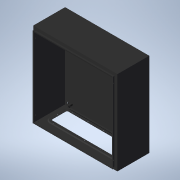
# Autodesk Inventor part: 1054.000(2)_P1
Saved by Autodesk Inventor 2021 (Build 250183000, 183)
## iProperties
Created: 2025-08-26
Part Number: 1054.000(2)_P1
Material: Generic
Catalog Web Link: www.cadenas.de
Description: AE 2.0 Gehaeuse-AE 2.0 Gehaeuse
Vendor: RITTAL
Document SubType Name: Modeling
Designer: psAdmin
Manufacturer: RITTAL
Mass: 1439.52 g
Surface Area: 19061.9 cm^2
Volume: 1439.52 cm^3
Density: 1 g/cm^3
Appearance: PSOLRGB-176-176-176
Category: PARTsolutions
Company: RITTAL
Title: 1054.000(2)_P1
Author: Cadenas PARTsolutions
Comments: AE 2.0 Gehaeuse
PSOL_IDENT_0: {$CADENAS_DATA/23d-libs/rittal/schaltschranksys/kompakt_schaltschr/parts_ae_2_0/gehaeuse_ae_2_0.prj}
PSOL_IDENT_1: ,190 {VTYP=3D},{NB=1054.000(2)_P1},{LINA=1054.000(2)_P1},{NN=AE 2.0 Gehaeuse},{DATE=25.07.2025 12:41
PSOL_IDENT_2: :23},{GEOMDATE=24.07.2025 05:50:00},{VERSION=},{LINEID=340},{WBVAR=DETAIL},{WBNUMERIC=DETAIL}  {NB=1
PSOL_IDENT_3: 054.000(2)_P1},{LINA=1054.000(2)_P1},{KT=DUMMY},{DETAIL=2},{BEZ1=Neues Kompaktgehäuse},{BEZ2=Stahlbl
PSOL_IDENT_4: ech},{BEZ3=eintürig},{TUER=1},{B=600},{H=600},{T=250},{F=550},{G=575},{B1=600},{BEST=1054.000},{B3=5
PSOL_IDENT_5: 60.000},{B4=470.000},{B5=498.000},{BB5=0.000},{H1=600},{H3=560.000},{H4=85.000},{H5=113.000},{HH5=4.
PSOL_IDENT_6: 000},{T5=93.500},{R1=31.000},{R2=8.000},{T1=250},{F1=550},{G1=575},{VERS3=0},{VERS=7},{CNSECLASS51=2
PSOL_IDENT_7: 7-18-01-02},{CNSECLASS70=27-18-01-01},{CNSECLASS80=27-18-01-01},{CNSETIM40=EC000261},{S=1.50},{W=600
PSOL_IDENT_8: .000},{W1=556.000},{W2=500.000},{HH=600.000},{HH1=556.000},{HH2=550.000},{HH3=475.000},{D=227.500},{
PSOL_IDENT_9: D1=245.100},{VERS1=1},{GEW=23,4},{CNSETIM80=EC000261},{CNSETIM90=EC000261},{CNSECLASS60=27-18-01-01}
PSOL_IDENT_10: ,{UNSPSC=31-26-15-02}
NB: 1054.000(2)_P1
NN: AE 2.0 Gehaeuse
NT: AE 2.0 Gehaeuse
NBSYN: $BEST.($DETAIL.)_P1
LINA: 1054.000(2)_P1
CATALOG: Rittal
DETAIL: niedrig
BEZ1: Neues Kompaktgehäuse
BEZ2: Stahlblech
BEZ3: eintürig
TUER: 1
B: 600
H: 600
T: 250
F: 550
G: 575
B1: 600
BEST: 1054.000
B3: 560
B4: 470
B5: 498
BB5: 0
H1: 600
H3: 560
H4: 85
H5: 113
HH5: 4
T5: 93.5
R1: 31
R2: 8
T1: 250
F1: 550
G1: 575
VERS3: 0
VERS: 7
CNSECLASS70: 27-18-01-01
CNSECLASS80: 27-18-01-01
S: 1.5
W: 600
W1: 556
W2: 500
HH: 600
HH1: 556
HH2: 550
HH3: 475
D: 227.5
D1: 245.1
VERS1: 1
GEW: 23,4
CNSETIM80: EC000261
CNSETIM90: EC000261
CNSECLASS60: 27-18-01-01
UNSPSC: 31-26-15-02
SUPPLIER: RITTAL
ARTICLENO: 1054.000(2)_P1
BOMINFO: 1054.000(2)_P1
CREATOR: CADENAS GmbH
Autodesk Inventor part; units mm, degrees
(part 1 of 2)
sketch "Sketch_1" plane through (0, 0, 0) normal (0, 1, 0) x (1, 0, 0)
  line L0 (-300, -102.5) -> (300, -102.5)
  line L1 (300, -102.5) -> (300, 125)
  line L2 (300, 125) -> (-300, 125)
  line L3 (-300, 125) -> (-300, -102.5)
  line L4 (-298.5, -101) -> (298.5, -101)
  line L5 (298.5, -101) -> (298.5, 123.5)
  line L6 (298.5, 123.5) -> (-298.5, 123.5)
  line L7 (-298.5, 123.5) -> (-298.5, -101)
  constraints: 16 end point
extrude "Extrusion1" add sketch "Sketch_1" along normal blind 600
sketch "Sketch_2" plane through (0, 0, 102.5) normal (0, 0, 1) x (1, 0, 0)
  line L0 (-281, 19) -> (281, 19)
  line L1 (281, 19) -> (281, 581)
  line L2 (281, 581) -> (-281, 581)
  line L3 (-281, 581) -> (-281, 19)
  constraints: 8 end point
extrude "Extrusion2" cut sketch "Sketch_2" against normal blind 1.5
sketch "Sketch_3" plane through (0, 0, 0) normal (1, 0, 0) x (0, 0, -1)
  line L0 (-102.5, 590) -> (-101, 590)
  line L1 (-101, 590) -> (-101, 598.5)
  line L2 (-101, 598.5) -> (123.5, 598.5)
  line L3 (123.5, 598.5) -> (123.5, 1.5)
  line L4 (123.5, 1.5) -> (-101, 1.5)
  line L5 (-101, 1.5) -> (-101, 10)
  line L6 (-101, 10) -> (-102.5, 10)
  line L7 (-102.5, 10) -> (-102.5, 0)
  line L8 (-102.5, 0) -> (125, 0)
  line L9 (125, 0) -> (125, 600)
  line L10 (125, 600) -> (-102.5, 600)
  line L11 (-102.5, 600) -> (-102.5, 590)
  constraints: 24 end point
extrude "Extrusion3" add sketch "Sketch_3" along normal mid plane 600
sketch "Sketch_48" plane through (0, 0, -125) normal (0, 0, 1) x (1, 0, 0)
  line L0 (-295.5, 595.5) -> (-295.5, 4.5)
  line L1 (-295.5, 4.5) -> (295.5, 4.5)
  line L2 (295.5, 4.5) -> (295.5, 595.5)
  line L3 (295.5, 595.5) -> (-295.5, 595.5)
  constraints: 8 end point
extrude "Extrusion4" cut sketch "Sketch_48" along normal blind 1.5
sketch "Sketch_49" plane through (0, 0, -125) normal (0, 0, 1) x (1, 0, 0)
  line L0 (-295.5, 595.5) -> (-295.5, 4.5)
  line L1 (-295.5, 4.5) -> (295.5, 4.5)
  line L2 (295.5, 4.5) -> (295.5, 595.5)
  line L3 (295.5, 595.5) -> (-295.5, 595.5)
  line L4 (268.5, 8.5) -> (291.5, 8.5)
  line L5 (291.5, 8.5) -> (291.5, 31.5)
  line L6 (291.5, 31.5) -> (268.5, 31.5)
  line L7 (268.5, 31.5) -> (268.5, 8.5)
  line L8 (268.5, 568.5) -> (291.5, 568.5)
  line L9 (291.5, 568.5) -> (291.5, 591.5)
  line L10 (291.5, 591.5) -> (268.5, 591.5)
  line L11 (268.5, 591.5) -> (268.5, 568.5)
  line L12 (-291.5, 8.5) -> (-268.5, 8.5)
  line L13 (-268.5, 8.5) -> (-268.5, 31.5)
  line L14 (-268.5, 31.5) -> (-291.5, 31.5)
  line L15 (-291.5, 31.5) -> (-291.5, 8.5)
  line L16 (-291.5, 568.5) -> (-268.5, 568.5)
  line L17 (-268.5, 568.5) -> (-268.5, 591.5)
  line L18 (-268.5, 591.5) -> (-291.5, 591.5)
  line L19 (-291.5, 591.5) -> (-291.5, 568.5)
  constraints: 40 end point
extrude "Extrusion5" add sketch "Sketch_49" along normal blind 1.5
sketch "Sketch_50" plane through (0, 20, 0) normal (0, 1, 0) x (1, 0, 0)
  line L0 (-291.5, 123.5) -> (-290.1732, 123.5)
  line L1 (-290.1732, 123.5) -> (-289.0185, 121.5)
  line L2 (-289.0185, 121.5) -> (-270.9815, 121.5)
  line L3 (-270.9815, 121.5) -> (-269.8268, 123.5)
  line L4 (-269.8268, 123.5) -> (-268.5, 123.5)
  line L5 (-268.5, 123.5) -> (-268.5, 125)
  line L6 (-268.5, 125) -> (-270, 125)
  line L7 (-270, 125) -> (-271.1547, 123)
  line L8 (-271.1547, 123) -> (-288.8453, 123)
  line L9 (-288.8453, 123) -> (-290, 125)
  line L10 (-290, 125) -> (-291.5, 125)
  line L11 (-291.5, 125) -> (-291.5, 123.5)
  constraints: 24 end point
extrude "Extrusion6" add sketch "Sketch_50" along normal mid plane 15.35
sketch "Sketch_51" plane through (0, 20, 0) normal (0, 1, 0) x (1, 0, 0)
  line L0 (268.5, 123.5) -> (269.8268, 123.5)
  line L1 (269.8268, 123.5) -> (270.9815, 121.5)
  line L2 (270.9815, 121.5) -> (289.0185, 121.5)
  line L3 (289.0185, 121.5) -> (290.1732, 123.5)
  line L4 (290.1732, 123.5) -> (291.5, 123.5)
  line L5 (291.5, 123.5) -> (291.5, 125)
  line L6 (291.5, 125) -> (290, 125)
  line L7 (290, 125) -> (288.8453, 123)
  line L8 (288.8453, 123) -> (271.1547, 123)
  line L9 (271.1547, 123) -> (270, 125)
  line L10 (270, 125) -> (268.5, 125)
  line L11 (268.5, 125) -> (268.5, 123.5)
  constraints: 24 end point
extrude "Extrusion7" add sketch "Sketch_51" along normal mid plane 15.35
sketch "Sketch_52" plane through (0, 27.675, 0) normal (0, 1, 0) x (1, 0, 0)
  line L0 (-272.325, 121.5) -> (-272.325, 123)
  line L1 (-272.325, 123) -> (-271.1547, 123)
  line L2 (-271.1547, 123) -> (-270, 125)
  line L3 (-270, 125) -> (-265.5, 125)
  line L4 (-265.5, 125) -> (-265.5, 123.5)
  line L5 (-265.5, 123.5) -> (-269.8268, 123.5)
  line L6 (-269.8268, 123.5) -> (-270.9815, 121.5)
  line L7 (-270.9815, 121.5) -> (-272.325, 121.5)
  line L8 (-272.325, 121.5) -> (-272.325, 123)
  constraints: 18 end point
revolve "Revolution1" add sketch "Sketch_52" angle 90 about axis through (-272.325, 27.675, -121.5) along (0, 0, 1)
sketch "Sketch_53" plane through (0, 27.675, 0) normal (0, 1, 0) x (1, 0, 0)
  line L0 (-287.675, 123) -> (-287.675, 121.5)
  line L1 (-287.675, 121.5) -> (-289.0185, 121.5)
  line L2 (-289.0185, 121.5) -> (-290.1732, 123.5)
  line L3 (-290.1732, 123.5) -> (-294.5, 123.5)
  line L4 (-294.5, 123.5) -> (-294.5, 125)
  line L5 (-294.5, 125) -> (-290, 125)
  line L6 (-290, 125) -> (-288.8453, 123)
  line L7 (-288.8453, 123) -> (-287.675, 123)
  line L8 (-287.675, 123) -> (-287.675, 121.5)
  constraints: 18 end point
revolve "Revolution2" add sketch "Sketch_53" angle 90 about axis through (-287.675, 27.675, -123) along (0, 0, -1)
sketch "Sketch_54" plane through (0, 27.675, 0) normal (0, 1, 0) x (1, 0, 0)
  line L0 (287.675, 121.5) -> (287.675, 123)
  line L1 (287.675, 123) -> (288.8453, 123)
  line L2 (288.8453, 123) -> (290, 125)
  line L3 (290, 125) -> (294.5, 125)
  line L4 (294.5, 125) -> (294.5, 123.5)
  line L5 (294.5, 123.5) -> (290.1732, 123.5)
  line L6 (290.1732, 123.5) -> (289.0185, 121.5)
  line L7 (289.0185, 121.5) -> (287.675, 121.5)
  line L8 (287.675, 121.5) -> (287.675, 123)
  constraints: 18 end point
revolve "Revolution3" add sketch "Sketch_54" angle 90 about axis through (287.675, 27.675, -121.5) along (0, 0, 1)
sketch "Sketch_55" plane through (0, 27.675, 0) normal (0, 1, 0) x (1, 0, 0)
  line L0 (272.325, 123) -> (272.325, 121.5)
  line L1 (272.325, 121.5) -> (270.9815, 121.5)
  line L2 (270.9815, 121.5) -> (269.8268, 123.5)
  line L3 (269.8268, 123.5) -> (265.5, 123.5)
  line L4 (265.5, 123.5) -> (265.5, 125)
  line L5 (265.5, 125) -> (270, 125)
  line L6 (270, 125) -> (271.1547, 123)
  line L7 (271.1547, 123) -> (272.325, 123)
  line L8 (272.325, 123) -> (272.325, 121.5)
  constraints: 18 end point
revolve "Revolution4" add sketch "Sketch_55" angle 90 about axis through (272.325, 27.675, -123) along (0, 0, -1)
sketch "Sketch_56" plane through (0, 12.325, 0) normal (0, 1, 0) x (1, 0, 0)
  line L0 (-272.325, 121.5) -> (-272.325, 123)
  line L1 (-272.325, 123) -> (-271.1547, 123)
  line L2 (-271.1547, 123) -> (-270, 125)
  line L3 (-270, 125) -> (-265.5, 125)
  line L4 (-265.5, 125) -> (-265.5, 123.5)
  line L5 (-265.5, 123.5) -> (-269.8268, 123.5)
  line L6 (-269.8268, 123.5) -> (-270.9815, 121.5)
  line L7 (-270.9815, 121.5) -> (-272.325, 121.5)
  line L8 (-272.325, 121.5) -> (-272.325, 123)
  constraints: 18 end point
revolve "Revolution5" add sketch "Sketch_56" angle 90 about axis through (-272.325, 12.325, -121.5) along (0, 0, -1)
sketch "Sketch_57" plane through (0, 12.325, 0) normal (0, 1, 0) x (1, 0, 0)
  line L0 (-287.675, 123) -> (-287.675, 121.5)
  line L1 (-287.675, 121.5) -> (-289.0185, 121.5)
  line L2 (-289.0185, 121.5) -> (-290.1732, 123.5)
  line L3 (-290.1732, 123.5) -> (-294.5, 123.5)
  line L4 (-294.5, 123.5) -> (-294.5, 125)
  line L5 (-294.5, 125) -> (-290, 125)
  line L6 (-290, 125) -> (-288.8453, 123)
  line L7 (-288.8453, 123) -> (-287.675, 123)
  line L8 (-287.675, 123) -> (-287.675, 121.5)
  constraints: 18 end point
revolve "Revolution6" add sketch "Sketch_57" angle 90 about axis through (-287.675, 12.325, -123) along (0, 0, 1)
sketch "Sketch_58" plane through (0, 12.325, 0) normal (0, 1, 0) x (1, 0, 0)
  line L0 (287.675, 121.5) -> (287.675, 123)
  line L1 (287.675, 123) -> (288.8453, 123)
  line L2 (288.8453, 123) -> (290, 125)
  line L3 (290, 125) -> (294.5, 125)
  line L4 (294.5, 125) -> (294.5, 123.5)
  line L5 (294.5, 123.5) -> (290.1732, 123.5)
  line L6 (290.1732, 123.5) -> (289.0185, 121.5)
  line L7 (289.0185, 121.5) -> (287.675, 121.5)
  line L8 (287.675, 121.5) -> (287.675, 123)
  constraints: 18 end point
revolve "Revolution7" add sketch "Sketch_58" angle 90 about axis through (287.675, 12.325, -121.5) along (0, 0, -1)
sketch "Sketch_59" plane through (0, 12.325, 0) normal (0, 1, 0) x (1, 0, 0)
  line L0 (272.325, 123) -> (272.325, 121.5)
  line L1 (272.325, 121.5) -> (270.9815, 121.5)
  line L2 (270.9815, 121.5) -> (269.8268, 123.5)
  line L3 (269.8268, 123.5) -> (265.5, 123.5)
  line L4 (265.5, 123.5) -> (265.5, 125)
  line L5 (265.5, 125) -> (270, 125)
  line L6 (270, 125) -> (271.1547, 123)
  line L7 (271.1547, 123) -> (272.325, 123)
  line L8 (272.325, 123) -> (272.325, 121.5)
  constraints: 18 end point
revolve "Revolution8" add sketch "Sketch_59" angle 90 about axis through (272.325, 12.325, -123) along (0, 0, 1)
sketch "Sketch_60" plane through (0, 580, 0) normal (0, 1, 0) x (1, 0, 0)
  line L0 (-291.5, 123.5) -> (-290.1732, 123.5)
  line L1 (-290.1732, 123.5) -> (-289.0185, 121.5)
  line L2 (-289.0185, 121.5) -> (-270.9815, 121.5)
  line L3 (-270.9815, 121.5) -> (-269.8268, 123.5)
  line L4 (-269.8268, 123.5) -> (-268.5, 123.5)
  line L5 (-268.5, 123.5) -> (-268.5, 125)
  line L6 (-268.5, 125) -> (-270, 125)
  line L7 (-270, 125) -> (-271.1547, 123)
  line L8 (-271.1547, 123) -> (-288.8453, 123)
  line L9 (-288.8453, 123) -> (-290, 125)
  line L10 (-290, 125) -> (-291.5, 125)
  line L11 (-291.5, 125) -> (-291.5, 123.5)
  constraints: 24 end point
extrude "Extrusion8" add sketch "Sketch_60" along normal mid plane 15.35
sketch "Sketch_61" plane through (0, 580, 0) normal (0, 1, 0) x (1, 0, 0)
  line L0 (268.5, 123.5) -> (269.8268, 123.5)
  line L1 (269.8268, 123.5) -> (270.9815, 121.5)
  line L2 (270.9815, 121.5) -> (289.0185, 121.5)
  line L3 (289.0185, 121.5) -> (290.1732, 123.5)
  line L4 (290.1732, 123.5) -> (291.5, 123.5)
  line L5 (291.5, 123.5) -> (291.5, 125)
  line L6 (291.5, 125) -> (290, 125)
  line L7 (290, 125) -> (288.8453, 123)
  line L8 (288.8453, 123) -> (271.1547, 123)
  line L9 (271.1547, 123) -> (270, 125)
  line L10 (270, 125) -> (268.5, 125)
  line L11 (268.5, 125) -> (268.5, 123.5)
  constraints: 24 end point
extrude "Extrusion9" add sketch "Sketch_61" along normal mid plane 15.35
sketch "Sketch_62" plane through (0, 587.675, 0) normal (0, 1, 0) x (1, 0, 0)
  line L0 (-272.325, 121.5) -> (-272.325, 123)
  line L1 (-272.325, 123) -> (-271.1547, 123)
  line L2 (-271.1547, 123) -> (-270, 125)
  line L3 (-270, 125) -> (-265.5, 125)
  line L4 (-265.5, 125) -> (-265.5, 123.5)
  line L5 (-265.5, 123.5) -> (-269.8268, 123.5)
  line L6 (-269.8268, 123.5) -> (-270.9815, 121.5)
  line L7 (-270.9815, 121.5) -> (-272.325, 121.5)
  line L8 (-272.325, 121.5) -> (-272.325, 123)
  constraints: 18 end point
revolve "Revolution9" add sketch "Sketch_62" angle 90 about axis through (-272.325, 587.675, -121.5) along (0, 0, 1)
sketch "Sketch_63" plane through (0, 587.675, 0) normal (0, 1, 0) x (1, 0, 0)
  line L0 (-287.675, 123) -> (-287.675, 121.5)
  line L1 (-287.675, 121.5) -> (-289.0185, 121.5)
  line L2 (-289.0185, 121.5) -> (-290.1732, 123.5)
  line L3 (-290.1732, 123.5) -> (-294.5, 123.5)
  line L4 (-294.5, 123.5) -> (-294.5, 125)
  line L5 (-294.5, 125) -> (-290, 125)
  line L6 (-290, 125) -> (-288.8453, 123)
  line L7 (-288.8453, 123) -> (-287.675, 123)
  line L8 (-287.675, 123) -> (-287.675, 121.5)
  constraints: 18 end point
revolve "Revolution10" add sketch "Sketch_63" angle 90 about axis through (-287.675, 587.675, -123) along (0, 0, -1)
sketch "Sketch_64" plane through (0, 587.675, 0) normal (0, 1, 0) x (1, 0, 0)
  line L0 (287.675, 121.5) -> (287.675, 123)
  line L1 (287.675, 123) -> (288.8453, 123)
  line L2 (288.8453, 123) -> (290, 125)
  line L3 (290, 125) -> (294.5, 125)
  line L4 (294.5, 125) -> (294.5, 123.5)
  line L5 (294.5, 123.5) -> (290.1732, 123.5)
  line L6 (290.1732, 123.5) -> (289.0185, 121.5)
  line L7 (289.0185, 121.5) -> (287.675, 121.5)
  line L8 (287.675, 121.5) -> (287.675, 123)
  constraints: 18 end point
revolve "Revolution11" add sketch "Sketch_64" angle 90 about axis through (287.675, 587.675, -121.5) along (0, 0, 1)
sketch "Sketch_65" plane through (0, 587.675, 0) normal (0, 1, 0) x (1, 0, 0)
  line L0 (272.325, 123) -> (272.325, 121.5)
  line L1 (272.325, 121.5) -> (270.9815, 121.5)
  line L2 (270.9815, 121.5) -> (269.8268, 123.5)
  line L3 (269.8268, 123.5) -> (265.5, 123.5)
  line L4 (265.5, 123.5) -> (265.5, 125)
  line L5 (265.5, 125) -> (270, 125)
  line L6 (270, 125) -> (271.1547, 123)
  line L7 (271.1547, 123) -> (272.325, 123)
  line L8 (272.325, 123) -> (272.325, 121.5)
  constraints: 18 end point
revolve "Revolution12" add sketch "Sketch_65" angle 90 about axis through (272.325, 587.675, -123) along (0, 0, -1)
sketch "Sketch_66" plane through (0, 572.325, 0) normal (0, 1, 0) x (1, 0, 0)
  line L0 (-272.325, 121.5) -> (-272.325, 123)
  line L1 (-272.325, 123) -> (-271.1547, 123)
  line L2 (-271.1547, 123) -> (-270, 125)
  line L3 (-270, 125) -> (-265.5, 125)
  line L4 (-265.5, 125) -> (-265.5, 123.5)
  line L5 (-265.5, 123.5) -> (-269.8268, 123.5)
  line L6 (-269.8268, 123.5) -> (-270.9815, 121.5)
  line L7 (-270.9815, 121.5) -> (-272.325, 121.5)
  line L8 (-272.325, 121.5) -> (-272.325, 123)
  constraints: 18 end point
revolve "Revolution13" add sketch "Sketch_66" angle 90 about axis through (-272.325, 572.325, -121.5) along (0, 0, -1)
sketch "Sketch_67" plane through (0, 572.325, 0) normal (0, 1, 0) x (1, 0, 0)
  line L0 (-287.675, 123) -> (-287.675, 121.5)
  line L1 (-287.675, 121.5) -> (-289.0185, 121.5)
  line L2 (-289.0185, 121.5) -> (-290.1732, 123.5)
  line L3 (-290.1732, 123.5) -> (-294.5, 123.5)
  line L4 (-294.5, 123.5) -> (-294.5, 125)
  line L5 (-294.5, 125) -> (-290, 125)
  line L6 (-290, 125) -> (-288.8453, 123)
  line L7 (-288.8453, 123) -> (-287.675, 123)
  line L8 (-287.675, 123) -> (-287.675, 121.5)
  constraints: 18 end point
revolve "Revolution14" add sketch "Sketch_67" angle 90 about axis through (-287.675, 572.325, -123) along (0, 0, 1)
sketch "Sketch_68" plane through (0, 572.325, 0) normal (0, 1, 0) x (1, 0, 0)
  line L0 (287.675, 121.5) -> (287.675, 123)
  line L1 (287.675, 123) -> (288.8453, 123)
  line L2 (288.8453, 123) -> (290, 125)
  line L3 (290, 125) -> (294.5, 125)
  line L4 (294.5, 125) -> (294.5, 123.5)
  line L5 (294.5, 123.5) -> (290.1732, 123.5)
  line L6 (290.1732, 123.5) -> (289.0185, 121.5)
  line L7 (289.0185, 121.5) -> (287.675, 121.5)
  line L8 (287.675, 121.5) -> (287.675, 123)
  constraints: 18 end point
revolve "Revolution15" add sketch "Sketch_68" angle 90 about axis through (287.675, 572.325, -121.5) along (0, 0, -1)
sketch "Sketch_69" plane through (0, 572.325, 0) normal (0, 1, 0) x (1, 0, 0)
  line L0 (272.325, 123) -> (272.325, 121.5)
  line L1 (272.325, 121.5) -> (270.9815, 121.5)
  line L2 (270.9815, 121.5) -> (269.8268, 123.5)
  line L3 (269.8268, 123.5) -> (265.5, 123.5)
  line L4 (265.5, 123.5) -> (265.5, 125)
  line L5 (265.5, 125) -> (270, 125)
  line L6 (270, 125) -> (271.1547, 123)
  line L7 (271.1547, 123) -> (272.325, 123)
  line L8 (272.325, 123) -> (272.325, 121.5)
  constraints: 18 end point
revolve "Revolution16" add sketch "Sketch_69" angle 90 about axis through (272.325, 572.325, -123) along (0, 0, 1)
sketch "Sketch_70" plane through (-280, 0, 0) normal (1, 0, 0) x (0, 0, -1)
  line L0 (121.5, 10.9815) -> (123.5, 9.8268)
  line L1 (123.5, 9.8268) -> (123.5, 8.5)
  line L2 (123.5, 8.5) -> (125, 8.5)
  line L3 (125, 8.5) -> (125, 10)
  line L4 (125, 10) -> (123, 11.1547)
  line L5 (123, 11.1547) -> (123, 28.8453)
  line L6 (123, 28.8453) -> (125, 30)
  line L7 (125, 30) -> (125, 31.5)
  line L8 (125, 31.5) -> (123.5, 31.5)
  line L9 (123.5, 31.5) -> (123.5, 30.1732)
  line L10 (123.5, 30.1732) -> (121.5, 29.0185)
  line L11 (121.5, 29.0185) -> (121.5, 10.9815)
  constraints: 24 end point
extrude "Extrusion10" add sketch "Sketch_70" along normal mid plane 15.35
sketch "Sketch_71" plane through (-280, 0, 0) normal (1, 0, 0) x (0, 0, -1)
  line L0 (121.5, 570.9815) -> (123.5, 569.8268)
  line L1 (123.5, 569.8268) -> (123.5, 568.5)
  line L2 (123.5, 568.5) -> (125, 568.5)
  line L3 (125, 568.5) -> (125, 570)
  line L4 (125, 570) -> (123, 571.1547)
  line L5 (123, 571.1547) -> (123, 588.8453)
  line L6 (123, 588.8453) -> (125, 590)
  line L7 (125, 590) -> (125, 591.5)
  line L8 (125, 591.5) -> (123.5, 591.5)
  line L9 (123.5, 591.5) -> (123.5, 590.1732)
  line L10 (123.5, 590.1732) -> (121.5, 589.0185)
  line L11 (121.5, 589.0185) -> (121.5, 570.9815)
  constraints: 24 end point
extrude "Extrusion11" add sketch "Sketch_71" along normal mid plane 15.35
sketch "Sketch_74" plane through (-280, 0, 0) normal (1, 0, 0) x (0, 0, -1)
  line L0 (124.5, 20) -> (121.5, 20)
  line L1 (121.5, 20) -> (121.5, 26.25)
  line L2 (121.5, 26.25) -> (123, 26.25)
  line L3 (123, 26.25) -> (123, 25.6)
  line L4 (123, 25.6) -> (124.5, 25.6)
  line L5 (124.5, 25.6) -> (124.5, 20)
  line L6 (124.5, 20) -> (121.5, 20)
  constraints: 14 end point
revolve "Revolution17" add sketch "Sketch_74" angle 360 about axis through (-280, 20, -124.5) along (0, 0, 1)
sketch "Sketch_75" plane through (-280, 0, 0) normal (1, 0, 0) x (0, 0, -1)
  line L0 (125, 20) -> (121, 20)
  line L1 (121, 20) -> (121, 25.625)
  line L2 (121, 25.625) -> (121.5, 25.625)
  line L3 (121.5, 25.625) -> (121.5, 24.625)
  line L4 (121.5, 24.625) -> (124.5, 24.625)
  line L5 (124.5, 24.625) -> (124.5, 25.625)
  line L6 (124.5, 25.625) -> (125, 25.625)
  line L7 (125, 25.625) -> (125, 20)
  line L8 (125, 20) -> (121, 20)
  constraints: 18 end point
revolve "Revolution18" cut sketch "Sketch_75" angle 360 about axis through (-280, 20, -125) along (0, 0, 1)
sketch "Sketch_76" plane through (-280, 0, 0) normal (1, 0, 0) x (0, 0, -1)
  line L0 (124.5, 580) -> (121.5, 580)
  line L1 (121.5, 580) -> (121.5, 586.25)
  line L2 (121.5, 586.25) -> (123, 586.25)
  line L3 (123, 586.25) -> (123, 585.6)
  line L4 (123, 585.6) -> (124.5, 585.6)
  line L5 (124.5, 585.6) -> (124.5, 580)
  line L6 (124.5, 580) -> (121.5, 580)
  constraints: 14 end point
revolve "Revolution19" add sketch "Sketch_76" angle 360 about axis through (-280, 580, -124.5) along (0, 0, 1)
sketch "Sketch_77" plane through (-280, 0, 0) normal (1, 0, 0) x (0, 0, -1)
  line L0 (125, 580) -> (121, 580)
  line L1 (121, 580) -> (121, 585.625)
  line L2 (121, 585.625) -> (121.5, 585.625)
  line L3 (121.5, 585.625) -> (121.5, 584.625)
  line L4 (121.5, 584.625) -> (124.5, 584.625)
  line L5 (124.5, 584.625) -> (124.5, 585.625)
  line L6 (124.5, 585.625) -> (125, 585.625)
  line L7 (125, 585.625) -> (125, 580)
  line L8 (125, 580) -> (121, 580)
  constraints: 18 end point
revolve "Revolution20" cut sketch "Sketch_77" angle 360 about axis through (-280, 580, -125) along (0, 0, 1)
sketch "Sketch_72" plane through (280, 0, 0) normal (1, 0, 0) x (0, 0, -1)
  line L0 (121.5, 10.9815) -> (123.5, 9.8268)
  line L1 (123.5, 9.8268) -> (123.5, 8.5)
  line L2 (123.5, 8.5) -> (125, 8.5)
  line L3 (125, 8.5) -> (125, 10)
  line L4 (125, 10) -> (123, 11.1547)
  line L5 (123, 11.1547) -> (123, 28.8453)
  line L6 (123, 28.8453) -> (125, 30)
  line L7 (125, 30) -> (125, 31.5)
  line L8 (125, 31.5) -> (123.5, 31.5)
  line L9 (123.5, 31.5) -> (123.5, 30.1732)
  line L10 (123.5, 30.1732) -> (121.5, 29.0185)
  line L11 (121.5, 29.0185) -> (121.5, 10.9815)
  constraints: 24 end point
extrude "Extrusion12" add sketch "Sketch_72" along normal mid plane 15.35
sketch "Sketch_73" plane through (280, 0, 0) normal (1, 0, 0) x (0, 0, -1)
  line L0 (121.5, 570.9815) -> (123.5, 569.8268)
  line L1 (123.5, 569.8268) -> (123.5, 568.5)
  line L2 (123.5, 568.5) -> (125, 568.5)
  line L3 (125, 568.5) -> (125, 570)
  line L4 (125, 570) -> (123, 571.1547)
  line L5 (123, 571.1547) -> (123, 588.8453)
  line L6 (123, 588.8453) -> (125, 590)
  line L7 (125, 590) -> (125, 591.5)
  line L8 (125, 591.5) -> (123.5, 591.5)
  line L9 (123.5, 591.5) -> (123.5, 590.1732)
  line L10 (123.5, 590.1732) -> (121.5, 589.0185)
  line L11 (121.5, 589.0185) -> (121.5, 570.9815)
  constraints: 24 end point
extrude "Extrusion13" add sketch "Sketch_73" along normal mid plane 15.35
sketch "Sketch_78" plane through (280, 0, 0) normal (1, 0, 0) x (0, 0, -1)
  line L0 (124.5, 20) -> (121.5, 20)
  line L1 (121.5, 20) -> (121.5, 26.25)
  line L2 (121.5, 26.25) -> (123, 26.25)
  line L3 (123, 26.25) -> (123, 25.6)
  line L4 (123, 25.6) -> (124.5, 25.6)
  line L5 (124.5, 25.6) -> (124.5, 20)
  line L6 (124.5, 20) -> (121.5, 20)
  constraints: 14 end point
revolve "Revolution21" add sketch "Sketch_78" angle 360 about axis through (280, 20, -124.5) along (0, 0, 1)
sketch "Sketch_79" plane through (280, 0, 0) normal (1, 0, 0) x (0, 0, -1)
  line L0 (125, 20) -> (121, 20)
  line L1 (121, 20) -> (121, 25.625)
  line L2 (121, 25.625) -> (121.5, 25.625)
  line L3 (121.5, 25.625) -> (121.5, 24.625)
  line L4 (121.5, 24.625) -> (124.5, 24.625)
  line L5 (124.5, 24.625) -> (124.5, 25.625)
  line L6 (124.5, 25.625) -> (125, 25.625)
  line L7 (125, 25.625) -> (125, 20)
  line L8 (125, 20) -> (121, 20)
  constraints: 18 end point
revolve "Revolution22" cut sketch "Sketch_79" angle 360 about axis through (280, 20, -125) along (0, 0, 1)
sketch "Sketch_80" plane through (280, 0, 0) normal (1, 0, 0) x (0, 0, -1)
  line L0 (124.5, 580) -> (121.5, 580)
  line L1 (121.5, 580) -> (121.5, 586.25)
  line L2 (121.5, 586.25) -> (123, 586.25)
  line L3 (123, 586.25) -> (123, 585.6)
  line L4 (123, 585.6) -> (124.5, 585.6)
  line L5 (124.5, 585.6) -> (124.5, 580)
  line L6 (124.5, 580) -> (121.5, 580)
  constraints: 14 end point
revolve "Revolution23" add sketch "Sketch_80" angle 360 about axis through (280, 580, -124.5) along (0, 0, 1)
sketch "Sketch_81" plane through (280, 0, 0) normal (1, 0, 0) x (0, 0, -1)
  line L0 (125, 580) -> (121, 580)
  line L1 (121, 580) -> (121, 585.625)
  line L2 (121, 585.625) -> (121.5, 585.625)
  line L3 (121.5, 585.625) -> (121.5, 584.625)
  line L4 (121.5, 584.625) -> (124.5, 584.625)
  line L5 (124.5, 584.625) -> (124.5, 585.625)
  line L6 (124.5, 585.625) -> (125, 585.625)
  line L7 (125, 585.625) -> (125, 580)
  line L8 (125, 580) -> (121, 580)
  constraints: 18 end point
revolve "Revolution24" cut sketch "Sketch_81" angle 360 about axis through (280, 580, -125) along (0, 0, 1)
sketch "Sketch_6" plane through (0, 0, 0) normal (1, 0, 0) x (0, 0, -1)
  line L0 (-120.1, 585.9693) -> (-119.4028, 578)
  line L1 (-119.4028, 578) -> (-101, 578)
  line L2 (-101, 578) -> (-101, 586.1)
  line L3 (-101, 586.1) -> (-118.6057, 586.1)
  line L4 (-118.6057, 586.1) -> (-120.1, 585.9693)
  constraints: 10 end point
extrude "Extrusion14" add sketch "Sketch_6" along normal mid plane 574.2
sketch "Sketch_7" plane through (0, 0, 0) normal (1, 0, 0) x (0, 0, -1)
  line L0 (-120.1, 14.0307) -> (-118.6057, 13.9)
  line L1 (-118.6057, 13.9) -> (-101, 13.9)
  line L2 (-101, 13.9) -> (-101, 22)
  line L3 (-101, 22) -> (-119.4028, 22)
  line L4 (-119.4028, 22) -> (-120.1, 14.0307)
  constraints: 10 end point
extrude "Extrusion15" add sketch "Sketch_7" along normal mid plane 574.2
sketch "Sketch_8" plane through (0, 300, 0) normal (0, 1, 0) x (1, 0, 0)
  line L0 (278, -119.4028) -> (285.9693, -120.1)
  line L1 (285.9693, -120.1) -> (286.1, -118.6057)
  line L2 (286.1, -118.6057) -> (286.1, -101)
  line L3 (286.1, -101) -> (278, -101)
  line L4 (278, -101) -> (278, -119.4028)
  constraints: 10 end point
extrude "Extrusion16" add sketch "Sketch_8" along normal mid plane 574.2
sketch "Sketch_9" plane through (0, 300, 0) normal (0, 1, 0) x (1, 0, 0)
  line L0 (-286.1, -118.6057) -> (-285.9693, -120.1)
  line L1 (-285.9693, -120.1) -> (-278, -119.4028)
  line L2 (-278, -119.4028) -> (-278, -101)
  line L3 (-278, -101) -> (-286.1, -101)
  line L4 (-286.1, -101) -> (-286.1, -118.6057)
  constraints: 10 end point
extrude "Extrusion17" add sketch "Sketch_9" along normal mid plane 574.2
sketch "Sketch_10" plane through (0, 300, 0) normal (0, 1, 0) x (1, 0, 0)
  line L0 (-287.6, -102.5) -> (-287.6, -123.1)
  line L1 (-287.6, -123.1) -> (287.6, -123.1)
  line L2 (287.6, -123.1) -> (287.6, -102.5)
  line L3 (287.6, -102.5) -> (279.5, -102.5)
  line L4 (279.5, -102.5) -> (279.5, -118.0283)
  line L5 (279.5, -118.0283) -> (286.1, -118.6057)
  line L6 (286.1, -118.6057) -> (285.9693, -120.1)
  line L7 (285.9693, -120.1) -> (-285.9693, -120.1)
  line L8 (-285.9693, -120.1) -> (-286.1, -118.6057)
  line L9 (-286.1, -118.6057) -> (-279.5, -118.0283)
  line L10 (-279.5, -118.0283) -> (-279.5, -102.5)
  line L11 (-279.5, -102.5) -> (-287.6, -102.5)
  constraints: 24 end point
extrude "Extrusion18" cut sketch "Sketch_10" along normal mid plane 572.2
sketch "Sketch_11" plane through (0, 0, 0) normal (1, 0, 0) x (0, 0, -1)
  line L0 (-123.1, 10.9) -> (-102.5, 10.9)
  line L1 (-102.5, 10.9) -> (-102.5, 20.5)
  line L2 (-102.5, 20.5) -> (-118.0283, 20.5)
  line L3 (-118.0283, 20.5) -> (-118.6057, 13.9)
  line L4 (-118.6057, 13.9) -> (-120.1, 14.0307)
  line L5 (-120.1, 14.0307) -> (-120.1, 585.9693)
  line L6 (-120.1, 585.9693) -> (-118.6057, 586.1)
  line L7 (-118.6057, 586.1) -> (-118.0283, 579.5)
  line L8 (-118.0283, 579.5) -> (-102.5, 579.5)
  line L9 (-102.5, 579.5) -> (-102.5, 589.1)
  line L10 (-102.5, 589.1) -> (-123.1, 589.1)
  line L11 (-123.1, 589.1) -> (-123.1, 10.9)
  constraints: 24 end point
extrude "Extrusion19" cut sketch "Sketch_11" along normal mid plane 572.2
sketch "Sketch_13" plane through (0, 575, 0) normal (0, 1, 0) x (1, 0, 0)
  line L0 (-250, 92.5) -> (-250, 123.5)
  line L1 (-250, 123.5) -> (-243.5, 123.5)
  line L2 (-243.5, 123.5) -> (-243.5, 122.5)
  line L3 (-243.5, 122.5) -> (-242.45, 122.5)
  line L4 (-242.45, 122.5) -> (-242.25, 122.3)
  line L5 (-242.25, 122.3) -> (-242.25, 113.3)
  arc A0 (-242.55, 113) -> (-242.25, 113.3) centre (-242.55, 113.3) ccw
  line L6 (-242.55, 113) -> (-242.25, 113)
  line L7 (-242.25, 113) -> (-242.25, 107.5)
  line L8 (-242.25, 107.5) -> (-246, 107.5)
  line L9 (-246, 107.5) -> (-246, 105)
  line L10 (-246, 105) -> (-241, 105)
  arc A1 (-240.8875, 102.5051) -> (-241, 105) centre (-241, 103.75) ccw
  line L11 (-240.8875, 102.5051) -> (-242.2, 102.3864)
  line L12 (-242.2, 102.3864) -> (-242.2, 97.3483)
  line L13 (-242.2, 97.3483) -> (-243.5, 97)
  line L14 (-243.5, 97) -> (-246, 97)
  line L15 (-246, 97) -> (-246, 93.267)
  line L16 (-246, 93.267) -> (-246.767, 92.5)
  line L17 (-246.767, 92.5) -> (-250, 92.5)
  line L18 (-250, 92.5) -> (-250, 123.5)
  constraints: 38 end point, 4 point on circle, 2 centre point
revolve "Revolution25" add sketch "Sketch_13" angle 360 about axis through (-250, 575, -92.5) along (0, 0, 1)
thread "Thread1" size "M8x1.25" class "6g" standard "ISO Metric profile" length 1.1716
sketch "Sketch_14" plane through (0, 575, 0) normal (0, 1, 0) x (1, 0, 0)
  line L0 (250, 92.5) -> (250, 123.5)
  line L1 (250, 123.5) -> (256.5, 123.5)
  line L2 (256.5, 123.5) -> (256.5, 122.5)
  line L3 (256.5, 122.5) -> (257.55, 122.5)
  line L4 (257.55, 122.5) -> (257.75, 122.3)
  line L5 (257.75, 122.3) -> (257.75, 113.3)
  arc A0 (257.45, 113) -> (257.75, 113.3) centre (257.45, 113.3) ccw
  line L6 (257.45, 113) -> (257.75, 113)
  line L7 (257.75, 113) -> (257.75, 107.5)
  line L8 (257.75, 107.5) -> (254, 107.5)
  line L9 (254, 107.5) -> (254, 105)
  line L10 (254, 105) -> (259, 105)
  arc A1 (259.1125, 102.5051) -> (259, 105) centre (259, 103.75) ccw
  line L11 (259.1125, 102.5051) -> (257.8, 102.3864)
  line L12 (257.8, 102.3864) -> (257.8, 97.3483)
  line L13 (257.8, 97.3483) -> (256.5, 97)
  line L14 (256.5, 97) -> (254, 97)
  line L15 (254, 97) -> (254, 93.267)
  line L16 (254, 93.267) -> (253.233, 92.5)
  line L17 (253.233, 92.5) -> (250, 92.5)
  line L18 (250, 92.5) -> (250, 123.5)
  constraints: 38 end point, 4 point on circle, 2 centre point
revolve "Revolution26" add sketch "Sketch_14" angle 360 about axis through (250, 575, -92.5) along (0, 0, 1)
thread "Thread2" size "M8x1.25" class "6g" standard "ISO Metric profile" length 1.1716
sketch "Sketch_15" plane through (0, 25, 0) normal (0, 1, 0) x (1, 0, 0)
  line L0 (-250, 92.5) -> (-250, 123.5)
  line L1 (-250, 123.5) -> (-243.5, 123.5)
  line L2 (-243.5, 123.5) -> (-243.5, 122.5)
  line L3 (-243.5, 122.5) -> (-242.45, 122.5)
  line L4 (-242.45, 122.5) -> (-242.25, 122.3)
  line L5 (-242.25, 122.3) -> (-242.25, 113.3)
  arc A0 (-242.55, 113) -> (-242.25, 113.3) centre (-242.55, 113.3) ccw
  line L6 (-242.55, 113) -> (-242.25, 113)
  line L7 (-242.25, 113) -> (-242.25, 107.5)
  line L8 (-242.25, 107.5) -> (-246, 107.5)
  line L9 (-246, 107.5) -> (-246, 105)
  line L10 (-246, 105) -> (-241, 105)
  arc A1 (-240.8875, 102.5051) -> (-241, 105) centre (-241, 103.75) ccw
  line L11 (-240.8875, 102.5051) -> (-242.2, 102.3864)
  line L12 (-242.2, 102.3864) -> (-242.2, 97.3483)
  line L13 (-242.2, 97.3483) -> (-243.5, 97)
  line L14 (-243.5, 97) -> (-246, 97)
  line L15 (-246, 97) -> (-246, 93.267)
  line L16 (-246, 93.267) -> (-246.767, 92.5)
  line L17 (-246.767, 92.5) -> (-250, 92.5)
  line L18 (-250, 92.5) -> (-250, 123.5)
  constraints: 38 end point, 4 point on circle, 2 centre point
revolve "Revolution27" add sketch "Sketch_15" angle 360 about axis through (-250, 25, -92.5) along (0, 0, 1)
thread "Thread3" size "M8x1.25" class "6g" standard "ISO Metric profile" length 1.1716
sketch "Sketch_16" plane through (0, 25, 0) normal (0, 1, 0) x (1, 0, 0)
  line L0 (250, 92.5) -> (250, 123.5)
  line L1 (250, 123.5) -> (256.5, 123.5)
  line L2 (256.5, 123.5) -> (256.5, 122.5)
  line L3 (256.5, 122.5) -> (257.55, 122.5)
  line L4 (257.55, 122.5) -> (257.75, 122.3)
  line L5 (257.75, 122.3) -> (257.75, 113.3)
  arc A0 (257.45, 113) -> (257.75, 113.3) centre (257.45, 113.3) ccw
  line L6 (257.45, 113) -> (257.75, 113)
  line L7 (257.75, 113) -> (257.75, 107.5)
  line L8 (257.75, 107.5) -> (254, 107.5)
  line L9 (254, 107.5) -> (254, 105)
  line L10 (254, 105) -> (259, 105)
  arc A1 (259.1125, 102.5051) -> (259, 105) centre (259, 103.75) ccw
  line L11 (259.1125, 102.5051) -> (257.8, 102.3864)
  line L12 (257.8, 102.3864) -> (257.8, 97.3483)
  line L13 (257.8, 97.3483) -> (256.5, 97)
  line L14 (256.5, 97) -> (254, 97)
  line L15 (254, 97) -> (254, 93.267)
  line L16 (254, 93.267) -> (253.233, 92.5)
  line L17 (253.233, 92.5) -> (250, 92.5)
  line L18 (250, 92.5) -> (250, 123.5)
  constraints: 38 end point, 4 point on circle, 2 centre point
revolve "Revolution28" add sketch "Sketch_16" angle 360 about axis through (250, 25, -92.5) along (0, 0, 1)
thread "Thread4" size "M8x1.25" class "6g" standard "ISO Metric profile" length 1.1716
sketch "Sketch_100" plane through (0, 0, -96.75) normal (0, 0, 1) x (1, 0, 0)
  line L0 (-297, 597) -> (-297, 3)
  line L1 (-297, 3) -> (297, 3)
  line L2 (297, 3) -> (297, 597)
  line L3 (297, 597) -> (-297, 597)
  line L4 (243.5, 571.2472) -> (250, 567.4944)
  line L5 (250, 567.4944) -> (256.5, 571.2472)
  line L6 (256.5, 571.2472) -> (256.5, 578.7528)
  line L7 (256.5, 578.7528) -> (250, 582.5056)
  line L8 (250, 582.5056) -> (243.5, 578.7528)
  line L9 (243.5, 578.7528) -> (243.5, 571.2472)
  line L10 (243.5, 21.2472) -> (250, 17.4944)
  line L11 (250, 17.4944) -> (256.5, 21.2472)
  line L12 (256.5, 21.2472) -> (256.5, 28.7528)
  line L13 (256.5, 28.7528) -> (250, 32.5056)
  line L14 (250, 32.5056) -> (243.5, 28.7528)
  line L15 (243.5, 28.7528) -> (243.5, 21.2472)
  line L16 (-6.5, 571.2472) -> (0, 567.4944)
  line L17 (0, 567.4944) -> (6.5, 571.2472)
  line L18 (6.5, 571.2472) -> (6.5, 578.7528)
  line L19 (6.5, 578.7528) -> (0, 582.5056)
  line L20 (0, 582.5056) -> (-6.5, 578.7528)
  line L21 (-6.5, 578.7528) -> (-6.5, 571.2472)
  line L22 (-6.5, 21.2472) -> (0, 17.4944)
  line L23 (0, 17.4944) -> (6.5, 21.2472)
  line L24 (6.5, 21.2472) -> (6.5, 28.7528)
  line L25 (6.5, 28.7528) -> (0, 32.5056)
  line L26 (0, 32.5056) -> (-6.5, 28.7528)
  line L27 (-6.5, 28.7528) -> (-6.5, 21.2472)
  line L28 (-256.5, 571.2472) -> (-250, 567.4944)
  line L29 (-250, 567.4944) -> (-243.5, 571.2472)
  line L30 (-243.5, 571.2472) -> (-243.5, 578.7528)
  line L31 (-243.5, 578.7528) -> (-250, 582.5056)
  line L32 (-250, 582.5056) -> (-256.5, 578.7528)
  line L33 (-256.5, 578.7528) -> (-256.5, 571.2472)
  line L34 (-256.5, 21.2472) -> (-250, 17.4944)
  line L35 (-250, 17.4944) -> (-243.5, 21.2472)
  line L36 (-243.5, 21.2472) -> (-243.5, 28.7528)
  line L37 (-243.5, 28.7528) -> (-250, 32.5056)
  line L38 (-250, 32.5056) -> (-256.5, 28.7528)
  line L39 (-256.5, 28.7528) -> (-256.5, 21.2472)
  constraints: 80 end point
extrude "Extrusion20" cut sketch "Sketch_100" against normal blind 6
sketch "Sketch_139" plane through (0, 25, 0) normal (0, 1, 0) x (1, 0, 0)
  line L0 (-250, 101.6814) -> (-250, 105)
  line L1 (-250, 105) -> (-241, 105)
  arc A0 (-240.8875, 102.5051) -> (-241, 105) centre (-241, 103.75) ccw
  line L2 (-240.8875, 102.5051) -> (-250, 101.6814)
  line L3 (-250, 101.6814) -> (-250, 105)
  constraints: 8 end point, 2 point on circle, 1 centre point
revolve "Revolution29" add sketch "Sketch_139" angle 360 about axis through (-250, 25, -101.6814) along (0, 0, 1)
sketch "Sketch_140" plane through (0, 25, 0) normal (0, 1, 0) x (1, 0, 0)
  line L0 (250, 101.6814) -> (250, 105)
  line L1 (250, 105) -> (259, 105)
  arc A0 (259.1125, 102.5051) -> (259, 105) centre (259, 103.75) ccw
  line L2 (259.1125, 102.5051) -> (250, 101.6814)
  line L3 (250, 101.6814) -> (250, 105)
  constraints: 8 end point, 2 point on circle, 1 centre point
revolve "Revolution30" add sketch "Sketch_140" angle 360 about axis through (250, 25, -101.6814) along (0, 0, 1)
sketch "Sketch51" plane through (279.5, 20.5, 118.0283) normal (1, 0, 0) x (0, 0, -1)
  point P0 (8.2783, 517)
hole "Hole1" at (279.5, 537.5, 109.75) direction (-1, 0, 0) diameter 6.5 depth 1.5
sketch "Sketch52" plane through (279.5, 20.5, 118.0283) normal (1, 0, 0) x (0, 0, -1)
  point P0 (8.2783, 42)
hole "Hole2" at (279.5, 62.5, 109.75) direction (-1, 0, 0) diameter 6.5 depth 1.5
sketch "Sketch53" plane through (-279.5, 20.5, 102.5) normal (-1, 0, 0) x (0, 0, 1)
  point P0 (7.25, 517)
hole "Hole3" at (-279.5, 537.5, 109.75) direction (1, 0, 0) diameter 6.5 depth 1.5
sketch "Sketch54" plane through (-279.5, 20.5, 102.5) normal (-1, 0, 0) x (0, 0, 1)
  point P0 (7.25, 42)
hole "Hole4" at (-279.5, 62.5, 109.75) direction (1, 0, 0) diameter 6.5 depth 1.5
sketch "Sketch_27" plane through (0, 0, 0) normal (0, 1, 0) x (1, 0, 0)
  line L0 (-295.5, -98) -> (295.5, -98)
  line L1 (295.5, -98) -> (295.5, 120.5)
  line L2 (295.5, 120.5) -> (-295.5, 120.5)
  line L3 (-295.5, 120.5) -> (-295.5, -98)
  constraints: 8 end point
extrude "Extrusion21" cut sketch "Sketch_27" along normal blind 1.5
sketch "Sketch_28" plane through (0, 0, 0) normal (0, 1, 0) x (1, 0, 0)
  line L0 (-295.5, -98) -> (295.5, -98)
  line L1 (295.5, -98) -> (295.5, 120.5)
  line L2 (295.5, 120.5) -> (-295.5, 120.5)
  line L3 (-295.5, 120.5) -> (-295.5, -98)
  arc A0 (-274, -11) -> (-235, -50) centre (-235, -11) ccw
  line L4 (-235, -50) -> (235, -50)
  arc A1 (235, -50) -> (274, -11) centre (235, -11) ccw
  line L5 (274, -11) -> (274, 74)
  arc A2 (274, 74) -> (235, 113) centre (235, 74) ccw
  line L6 (235, 113) -> (-235, 113)
  arc A3 (-235, 113) -> (-274, 74) centre (-235, 74) ccw
  line L7 (-274, 74) -> (-274, -11)
  circle A4 centre (-283.5, -86) radius 8
  constraints: 16 end point, 8 point on circle, 5 centre point
extrude "Extrusion22" add sketch "Sketch_28" along normal blind 1.5
sketch "Sketch_29" plane through (0, 0, 0) normal (1, 0, 0) x (0, 0, -1)
  line L0 (88, 4) -> (104.5981, 4)
  line L1 (104.5981, 4) -> (111.5263, 0)
  line L2 (111.5263, 0) -> (113, 0)
  line L3 (113, 0) -> (113, 1.5)
  line L4 (113, 1.5) -> (111.9282, 1.5)
  line L5 (111.9282, 1.5) -> (105, 5.5)
  line L6 (105, 5.5) -> (88, 5.5)
  line L7 (88, 5.5) -> (88, 4)
  constraints: 16 end point
extrude "Extrusion23" add sketch "Sketch_29" along normal mid plane 470
sketch "Sketch_30" plane through (0, 0, 0) normal (1, 0, 0) x (0, 0, -1)
  line L0 (-50, 0) -> (-48.5263, 0)
  line L1 (-48.5263, 0) -> (-41.5981, 4)
  line L2 (-41.5981, 4) -> (-25, 4)
  line L3 (-25, 4) -> (-25, 5.5)
  line L4 (-25, 5.5) -> (-42, 5.5)
  line L5 (-42, 5.5) -> (-48.9282, 1.5)
  line L6 (-48.9282, 1.5) -> (-50, 1.5)
  line L7 (-50, 1.5) -> (-50, 0)
  constraints: 16 end point
extrude "Extrusion24" add sketch "Sketch_30" along normal mid plane 470
sketch "Sketch_31" plane through (235, 0, 0) normal (1, 0, 0) x (0, 0, -1)
  line L0 (74, 4) -> (74, 5.5)
  line L1 (88, 4) -> (104.5981, 4)
  line L2 (104.5981, 4) -> (111.5263, 0)
  line L3 (111.5263, 0) -> (115, 0)
  line L4 (115, 0) -> (115, 1.5)
  line L5 (115, 1.5) -> (111.9282, 1.5)
  line L6 (111.9282, 1.5) -> (105, 5.5)
  line L7 (105, 5.5) -> (88, 5.5)
  line L8 (88, 5.5) -> (88, 4)
  constraints: 18 end point
revolve "Revolution31" add sketch "Sketch_31" angle 90 about axis through (235, 4, -74) along (0, -1, 0)
sketch "Sketch_32" plane through (235, 0, 0) normal (1, 0, 0) x (0, 0, -1)
  line L0 (-11, 5.5) -> (-11, 4)
  line L1 (-52, 0) -> (-48.5263, 0)
  line L2 (-48.5263, 0) -> (-41.5981, 4)
  line L3 (-41.5981, 4) -> (-25, 4)
  line L4 (-25, 4) -> (-25, 5.5)
  line L5 (-25, 5.5) -> (-42, 5.5)
  line L6 (-42, 5.5) -> (-48.9282, 1.5)
  line L7 (-48.9282, 1.5) -> (-52, 1.5)
  line L8 (-52, 1.5) -> (-52, 0)
  constraints: 18 end point
revolve "Revolution32" add sketch "Sketch_32" angle 90 about axis through (235, 5.5, 11) along (0, 1, 0)
sketch "Sketch_33" plane through (-235, 0, 0) normal (1, 0, 0) x (0, 0, -1)
  line L0 (74, 4) -> (74, 5.5)
  line L1 (88, 4) -> (104.5981, 4)
  line L2 (104.5981, 4) -> (111.5263, 0)
  line L3 (111.5263, 0) -> (115, 0)
  line L4 (115, 0) -> (115, 1.5)
  line L5 (115, 1.5) -> (111.9282, 1.5)
  line L6 (111.9282, 1.5) -> (105, 5.5)
  line L7 (105, 5.5) -> (88, 5.5)
  line L8 (88, 5.5) -> (88, 4)
  constraints: 18 end point
revolve "Revolution33" add sketch "Sketch_33" angle 90 about axis through (-235, 4, -74) along (0, 1, 0)
sketch "Sketch_34" plane through (-235, 0, 0) normal (1, 0, 0) x (0, 0, -1)
  line L0 (-11, 5.5) -> (-11, 4)
  line L1 (-52, 0) -> (-48.5263, 0)
  line L2 (-48.5263, 0) -> (-41.5981, 4)
  line L3 (-41.5981, 4) -> (-25, 4)
  line L4 (-25, 4) -> (-25, 5.5)
  line L5 (-25, 5.5) -> (-42, 5.5)
  line L6 (-42, 5.5) -> (-48.9282, 1.5)
  line L7 (-48.9282, 1.5) -> (-52, 1.5)
  line L8 (-52, 1.5) -> (-52, 0)
  constraints: 18 end point
revolve "Revolution34" add sketch "Sketch_34" angle 90 about axis through (-235, 5.5, 11) along (0, -1, 0)
sketch "Sketch_35" plane through (0, 0, -31.5) normal (0, 0, 1) x (1, 0, 0)
  line L0 (249, 4) -> (265.5981, 4)
  line L1 (265.5981, 4) -> (272.5263, 0)
  line L2 (272.5263, 0) -> (274, 0)
  line L3 (274, 0) -> (274, 1.5)
  line L4 (274, 1.5) -> (272.9282, 1.5)
  line L5 (272.9282, 1.5) -> (266, 5.5)
  line L6 (266, 5.5) -> (249, 5.5)
  line L7 (249, 5.5) -> (249, 4)
  constraints: 16 end point
extrude "Extrusion25" add sketch "Sketch_35" along normal mid plane 85
sketch "Sketch_36" plane through (0, 0, -31.5) normal (0, 0, 1) x (1, 0, 0)
  line L0 (-274, 0) -> (-272.5263, 0)
  line L1 (-272.5263, 0) -> (-265.5981, 4)
  line L2 (-265.5981, 4) -> (-249, 4)
  line L3 (-249, 4) -> (-249, 5.5)
  line L4 (-249, 5.5) -> (-266, 5.5)
  line L5 (-266, 5.5) -> (-272.9282, 1.5)
  line L6 (-272.9282, 1.5) -> (-274, 1.5)
  line L7 (-274, 1.5) -> (-274, 0)
  constraints: 16 end point
extrude "Extrusion26" add sketch "Sketch_36" along normal mid plane 85
sketch "Sketch_37" plane through (0, 5.5, 0) normal (0, 1, 0) x (1, 0, 0)
  arc A0 (-264, -12) -> (-236, -40) centre (-236, -12) ccw
  line L0 (-236, -40) -> (236, -40)
  arc A1 (236, -40) -> (264, -12) centre (236, -12) ccw
  line L1 (264, -12) -> (264, 75)
  arc A2 (264, 75) -> (236, 103) centre (236, 75) ccw
  line L2 (236, 103) -> (-236, 103)
  arc A3 (-236, 103) -> (-264, 75) centre (-236, 75) ccw
  line L3 (-264, 75) -> (-264, -12)
  constraints: 8 end point, 8 point on circle, 4 centre point
extrude "Extrusion27" cut sketch "Sketch_37" against normal blind 1.5
sketch "Sketch_87" plane through (0, 5.5, 0) normal (0, 1, 0) x (1, 0, 0)
  arc A0 (-264, -12) -> (-236, -40) centre (-236, -12) ccw
  line L0 (-236, -40) -> (236, -40)
  arc A1 (236, -40) -> (264, -12) centre (236, -12) ccw
  line L1 (264, -12) -> (264, 75)
  arc A2 (264, 75) -> (236, 103) centre (236, 75) ccw
  line L2 (236, 103) -> (-236, 103)
  arc A3 (-236, 103) -> (-264, 75) centre (-236, 75) ccw
  line L3 (-264, 75) -> (-264, -12)
  circle A4 centre (259, 31.5) radius 2.2
  circle A5 centre (220, -35) radius 2.2
  circle A6 centre (220, 98) radius 2.2
  circle A7 centre (110, -35) radius 2.2
  circle A8 centre (110, 98) radius 2.2
  circle A9 centre (0, -35) radius 2.2
  circle A10 centre (0, 98) radius 2.2
  circle A11 centre (-110, -35) radius 2.2
  circle A12 centre (-110, 98) radius 2.2
  circle A13 centre (-220, -35) radius 2.2
  circle A14 centre (-220, 98) radius 2.2
  arc A15 (-249, -17) -> (-241, -25) centre (-241, -17) ccw
  line L4 (-241, -25) -> (241, -25)
  arc A16 (241, -25) -> (249, -17) centre (241, -17) ccw
  line L5 (249, -17) -> (249, 80)
  arc A17 (249, 80) -> (241, 88) centre (241, 80) ccw
  line L6 (241, 88) -> (-241, 88)
  arc A18 (-241, 88) -> (-249, 80) centre (-241, 80) ccw
  line L7 (-249, 80) -> (-249, -17)
  circle A19 centre (-259, 31.5) radius 2.2
  constraints: 20 centre point, 16 end point, 16 point on circle
extrude "Extrusion28" add sketch "Sketch_87" against normal blind 1.5
sketch "Sketch_106" plane through (0, 0, 32.5) normal (0, 0, 1) x (1, 0, 0)
  line L0 (298.5, 17.5) -> (278.1, 17.5)
  line L1 (278.1, 17.5) -> (278.1, 21.5)
  line L2 (278.1, 21.5) -> (293.1, 21.5)
  line L3 (293.1, 21.5) -> (293.1, 24.5)
  line L4 (293.1, 24.5) -> (298.5, 24.5)
  line L5 (298.5, 24.5) -> (298.5, 17.5)
  line L6 (298.5, 17.5) -> (278.1, 17.5)
  constraints: 14 end point
revolve "Revolution35" add sketch "Sketch_106" angle 360 about axis through (298.5, 17.5, 32.5) along (-1, 0, 0)
ref_plane "FP1_XY" through (0, -0.5, -31.5) normal (0, 1, 0) x (1, 0, 0)
ref_plane "FP1_YZ" through (0, -0.5, -31.5) normal (1, 0, 0) x (0, 0, -1)
ref_plane "FP1_ZX" through (0, -0.5, -31.5) normal (0, 0, -1) x (0, 1, 0)
ref_plane "FP2_XY" through (0, -0.5, -31.5) normal (0, 1, 0) x (1, 0, 0)
ref_plane "FP2_YZ" through (0, -0.5, -31.5) normal (1, 0, 0) x (0, 0, -1)
ref_plane "FP2_ZX" through (0, -0.5, -31.5) normal (0, 0, -1) x (0, 1, 0)
ref_plane "GEHAEUSE_XY" through (0, 300, -125) normal (0, 1, 0) x (1, 0, 0)
ref_plane "GEHAEUSE_YZ" through (0, 300, -125) normal (1, 0, 0) x (0, 0, -1)
ref_plane "GEHAEUSE_ZX" through (0, 300, -125) normal (0, 0, -1) x (0, 1, 0)
ref_plane "MP_XY" through (0, 25, -105) normal (0, 0, -1) x (1, 0, 0)
ref_plane "MP_YZ" through (0, 25, -105) normal (1, 0, 0) x (0, -1, 0)
ref_plane "MP_ZX" through (0, 25, -105) normal (0, -1, 0) x (0, 0, -1)
ref_plane "REVIT_XY" through (0, 0, -125) normal (0, 0, -1) x (-1, 0, 0)
ref_plane "REVIT_YZ" through (0, 0, -125) normal (-1, 0, 0) x (0, 1, 0)
ref_plane "REVIT_ZX" through (0, 0, -125) normal (0, 1, 0) x (0, 0, -1)
ref_plane "SCLM_XY" through (-279.5, 300, 109.75) normal (1, 0, 0) x (0, 0, -1)
ref_plane "SCLM_YZ" through (-279.5, 300, 109.75) normal (0, 0, -1) x (0, 1, 0)
ref_plane "SCLM_ZX" through (-279.5, 300, 109.75) normal (0, 1, 0) x (1, 0, 0)
ref_plane "SCLO_XY" through (-279.5, 537.5, 109.75) normal (1, 0, 0) x (0, 0, -1)
ref_plane "SCLO_YZ" through (-279.5, 537.5, 109.75) normal (0, 0, -1) x (0, 1, 0)
ref_plane "SCLO_ZX" through (-279.5, 537.5, 109.75) normal (0, 1, 0) x (1, 0, 0)
ref_plane "SCLU_XY" through (-279.5, 62.5, 109.75) normal (1, 0, 0) x (0, 0, -1)
ref_plane "SCLU_YZ" through (-279.5, 62.5, 109.75) normal (0, 0, -1) x (0, 1, 0)
ref_plane "SCLU_ZX" through (-279.5, 62.5, 109.75) normal (0, 1, 0) x (1, 0, 0)
ref_plane "SCRM_XY" through (279.5, 300, 109.75) normal (-1, 0, 0) x (0, 0, -1)
ref_plane "SCRM_YZ" through (279.5, 300, 109.75) normal (0, 0, -1) x (0, -1, 0)
ref_plane "SCRM_ZX" through (279.5, 300, 109.75) normal (0, -1, 0) x (-1, 0, 0)
ref_plane "SCRO_XY" through (279.5, 537.5, 109.75) normal (-1, 0, 0) x (0, 0, -1)
ref_plane "SCRO_YZ" through (279.5, 537.5, 109.75) normal (0, 0, -1) x (0, -1, 0)
ref_plane "SCRO_ZX" through (279.5, 537.5, 109.75) normal (0, -1, 0) x (-1, 0, 0)
ref_plane "SCRU_XY" through (279.5, 62.5, 109.75) normal (-1, 0, 0) x (0, 0, -1)
ref_plane "SCRU_YZ" through (279.5, 62.5, 109.75) normal (0, 0, -1) x (0, -1, 0)
ref_plane "SCRU_ZX" through (279.5, 62.5, 109.75) normal (0, -1, 0) x (-1, 0, 0)
ref_plane "to_Abst_tzung_L_XY" through (-250, 25, -96.75) normal (0, 0, 1) x (1, 0, 0)
ref_plane "to_Abst_tzung_L_YZ" through (-250, 25, -96.75) normal (1, 0, 0) x (0, 1, 0)
ref_plane "to_Abst_tzung_L_ZX" through (-250, 25, -96.75) normal (0, 1, 0) x (0, 0, 1)
ref_plane "to_Abst_tzung_R_XY" through (250, 25, -96.75) normal (0, 0, 1) x (1, 0, 0)
ref_plane "to_Abst_tzung_R_YZ" through (250, 25, -96.75) normal (1, 0, 0) x (0, 1, 0)
ref_plane "to_Abst_tzung_R_ZX" through (250, 25, -96.75) normal (0, 1, 0) x (0, 0, 1)
ref_plane "to_Cap_1_XY" through (280, 20, -125) normal (0, 0, 1) x (1, 0, 0)
ref_plane "to_Cap_1_YZ" through (280, 20, -125) normal (1, 0, 0) x (0, 1, 0)
ref_plane "to_Cap_1_ZX" through (280, 20, -125) normal (0, 1, 0) x (0, 0, 1)
ref_plane "to_Cap_2_XY" through (-280, 20, -125) normal (0, 0, 1) x (1, 0, 0)
ref_plane "to_Cap_2_YZ" through (-280, 20, -125) normal (1, 0, 0) x (0, 1, 0)
ref_plane "to_Cap_2_ZX" through (-280, 20, -125) normal (0, 1, 0) x (0, 0, 1)
ref_plane "to_Cap_3_XY" through (280, 580, -125) normal (0, 0, 1) x (1, 0, 0)
ref_plane "to_Cap_3_YZ" through (280, 580, -125) normal (1, 0, 0) x (0, 1, 0)
ref_plane "to_Cap_3_ZX" through (280, 580, -125) normal (0, 1, 0) x (0, 0, 1)
ref_plane "to_Cap_4_XY" through (-280, 580, -125) normal (0, 0, 1) x (1, 0, 0)
ref_plane "to_Cap_4_YZ" through (-280, 580, -125) normal (1, 0, 0) x (0, 1, 0)
ref_plane "to_Cap_4_ZX" through (-280, 580, -125) normal (0, 1, 0) x (0, 0, 1)
ref_plane "to_Plug_XY" through (-283.5, 0, 86) normal (0, 1, 0) x (1, 0, 0)
ref_plane "to_Plug_YZ" through (-283.5, 0, 86) normal (1, 0, 0) x (0, 0, -1)
ref_plane "to_Plug_ZX" through (-283.5, 0, 86) normal (0, 0, -1) x (0, 1, 0)
ref_plane "to_Plug_3_XY" through (250, 600, -3.5) normal (0, 1, 0) x (1, 0, 0)
ref_plane "to_Plug_3_YZ" through (250, 600, -3.5) normal (1, 0, 0) x (0, 0, -1)
ref_plane "to_Plug_3_ZX" through (250, 600, -3.5) normal (0, 0, -1) x (0, 1, 0)
ref_plane "to_Plug_4_XY" through (-250, 600, -3.5) normal (0, 1, 0) x (1, 0, 0)
ref_plane "to_Plug_4_YZ" through (-250, 600, -3.5) normal (1, 0, 0) x (0, 0, -1)
ref_plane "to_Plug_4_ZX" through (-250, 600, -3.5) normal (0, 0, -1) x (0, 1, 0)
ref_plane "to_Plug_1_1_XY" through (255, 0, -80) normal (0, 1, 0) x (1, 0, 0)
ref_plane "to_Plug_1_1_YZ" through (255, 0, -80) normal (1, 0, 0) x (0, 0, -1)
ref_plane "to_Plug_1_1_ZX" through (255, 0, -80) normal (0, 0, -1) x (0, 1, 0)